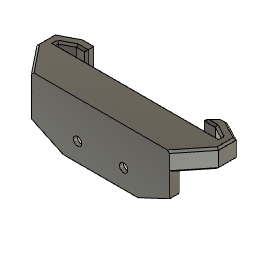
model (Autodesk Fusion 360 design; units mm, degrees)
Autodesk Fusion 360 part; units mm, degrees
sketch "saddle profile" plane through (0, 0, 0) normal (0, 0, 1) x (1, 0, 0) in component "hook"
  line L0 (0, 0) -> (0, 1.45)
  line L1 (0, 1.45) -> (4.9, 4)
  line L2 (4.9, 4) -> (11.5, 4)
  line L3 (11.5, 4) -> (11.5, 8)
  line L4 (11.5, 8) -> (37, 8)
  line L5 (37, 0) -> (0, 0)
  line L6 (37, 8) -> (37, 0) construction
  line L7 (74, 0) -> (74, 1.45)
  line L8 (74, 1.45) -> (69.1, 4)
  line L9 (69.1, 4) -> (62.5, 4)
  line L10 (62.5, 4) -> (62.5, 8)
  line L11 (62.5, 8) -> (37, 8)
  line L12 (37, 0) -> (74, 0)
  line L13 (0, 0) -> (0, -19.5) construction
  line L14 (0, -19.5) -> (74, -19.5) construction
  line L15 (74, -19.5) -> (74, 0) construction
  dimension "d7" = 1.45
  dimension "d8" = 6.6
  dimension "d9" = 4
  dimension "d10" = 11.5
  dimension "d11" = 4
  dimension "d12" = 37
  dimension "d13" = 19.5
  constraint coincident L0.start L5.end
  constraint vertical L0
  constraint perpendicular L0 L2
  constraint perpendicular L2 L3
  constraint perpendicular L3 L4
  constraint perpendicular L0 L5
  constraint perpendicular L5 L6
  constraint symmetric L0.start L6 L7.start
  constraint symmetric L0.end L6 L7.end
  constraint symmetric L1.end L6 L8.end
  constraint symmetric L2.end L6 L9.end
  constraint symmetric L3.end L6 L10.end
  constraint symmetric L4.end L6 L11.end
  constraint symmetric L5.start L6 L12.start
  constraint perpendicular L5 L13
  constraint perpendicular L0 L14
  constraint perpendicular L12 L15
  measures "d7" distance of L0.start L0.end
  measures "d8" distance of L1.end L2.end
  measures "d9" distance of L2 L5
  measures "d10" distance of L0 L3
  measures "d11" distance of L2.end L3.end
  measures "d12" distance of L5.start L0.start
  measures "d13" distance of L0.start L13.end
sketch "mount profile" plane through (0, 0, 0) normal (0, 0, 1) x (1, 0, 0) in component "hook"
  line L0 (-11.6, 4.4845) -> (-11.6, -5)
  line L1 (0, -19.5) -> (74, -19.5)
  line L2 (-6.6, 1.45) -> (-0.1627, 4.8)
  line L3 (5.0442, 9.8) -> (-1.3859, 9.8)
  line L4 (-1.3859, 9.8) -> (-11.6, 4.4845)
  line L5 (-0.1627, 4.8) -> (5.0442, 4.8)
  line L6 (5.0442, 4.8) -> (5.0442, 9.8)
  line L7 (0, 1.45) -> (4.9, 4)
  line L8 (75.3859, 9.8) -> (72.2442, 9.8)
  line L9 (74.1627, 4.8) -> (67.2442, 4.8)
  line L10 (67.2442, 4.8) -> (72.2442, 9.8)
  line L11 (85.6, -5) -> (85.6, 4.4845)
  line L12 (80.6, 0) -> (-6.6, 0)
  line L13 (-6.6, 0) -> (-6.6, 1.45)
  line L14 (80.6, 0) -> (80.6, 1.45)
  line L15 (80.6, 1.45) -> (74.1627, 4.8)
  line L16 (-3.3814, 3.125) -> (-5.6896, 7.5603) construction
  line L17 (85.6, 4.4845) -> (75.3859, 9.8)
  line L18 (77.3814, 3.125) -> (79.6896, 7.5603) construction
  line L19 (85.6, 0.725) -> (80.6, 0.725) construction
  line L20 (-6.6, 0.725) -> (-11.6, 0.725) construction
  line L21 (85.6, -5) -> (74, -19.5)
  line L22 (-11.6, -5) -> (0, -19.5)
  line L23 (85.6, -5) -> (-11.6, -5) construction
  line L24 (37, 0) -> (37, -5) construction
  line L25 (74, -19.5) -> (74, -13.5)
  line L26 (74, -13.5) -> (0, -13.5)
  line L27 (0, -13.5) -> (0, -19.5)
  point P0 (74, 0)
  point P1 (74, -19.5)
  point P2 (0, -19.5)
  dimension "d16" = 74
  dimension "d17" = 1.45
  dimension "d19" = 4.8
  dimension "d20" = 62.2
  dimension "d22" = 6.6
  dimension "d23" = 45
  dimension "d24" = 6.6
  dimension "d25" = 5
  dimension "d26" = 19.5
  dimension "d29" = 6
  dimension "d47" = 5.2069
  constraint vertical L0
  constraint horizontal L1
  constraint parallel L1 L5
  constraint perpendicular L1 L6
  constraint coincident L3.start L6.end
  constraint parallel L2 L7
  constraint coincident L8.end L10.end
  constraint perpendicular L8 L11
  constraint perpendicular L12 L13
  constraint coincident L2.start L13.end
  constraint horizontal L12
  constraint coincident origin L12
  constraint perpendicular L12 L14
  constraint parallel L9 L12
  constraint collinear L5 L9
  constraint equal L13 L14
  constraint equal L2 L15
  constraint parallel L2 L4
  constraint parallel L3 L5
  constraint midpoint L2 L16.start
  constraint coincident L4 L16.end
  constraint perpendicular L4 L16
  constraint equal L6 L16
  constraint collinear L3 L8
  constraint parallel L15 L17
  constraint midpoint L15 L18.start
  constraint coincident L17 L18.end
  constraint perpendicular L17 L18
  constraint equal L6 L18
  constraint coincident L11 L19.start
  constraint midpoint L14 L19.end
  constraint perpendicular L11 L19
  constraint equal L6 L19
  constraint midpoint L13 L20.start
  constraint coincident L0 L20.end
  constraint perpendicular L0 L20
  constraint equal L6 L20
  constraint coincident P1 L1.end
  constraint coincident P2 L1.start
  constraint horizontal L23
  constraint midpoint L12 L24.start
  constraint midpoint L23 L24.end
  constraint equal L6 L24
  constraint perpendicular L1 L25
  constraint perpendicular L25 L26
  constraint perpendicular L1 L27
  measures "d16" distance of L9.end L12.end
  measures "d17" distance of L12.end L2.start
  measures "d19" distance of L9 L12
  measures "d20" distance of L5.end L9.end
  measures "d22" distance of origin L12.end
  measures "d23" angle of L9 L10
  measures "d24" distance of L12.start P0
  measures "d25" distance of L16.start L16.end
  measures "d26" distance of L1 L12
  measures "d29" distance of L1 L26
  measures "d47" distance of L2.end L5.end
extrude "Extrude2" add sketch "mount profile" along normal blind 10 in component "hook"
sketch "mount" plane through (0, -19.5, 0) normal (0, -1, 0) x (1, 0, 0) in component "hook"
  line L0 (0, 0) -> (74, 0)
  line L1 (74, 0) -> (74, 10)
  line L2 (74, 10) -> (0, 10)
  line L3 (0, 10) -> (0, 0)
  line L4 (0, 0) -> (0, -12)
  line L5 (0, -12) -> (17, -20)
  line L6 (17, -20) -> (57, -20)
  line L7 (57, -20) -> (74, -12)
  line L8 (74, -12) -> (74, 0)
  circle A0 centre (24.6397, -10) radius 6.25 construction
  circle A1 centre (49.3603, -10) radius 6.25 construction
  circle A2 centre (24.6397, -10) radius 2.25
  circle A3 centre (49.3603, -10) radius 2.25
  line L9 (24.6397, -10) -> (49.3603, -10) construction
  line L10 (24.6397, -10) -> (0, -12) construction
  line L11 (49.3603, -10) -> (74, -12) construction
  line L12 (42, 0) -> (42, -20)
  line L13 (32, 0) -> (32, -20)
  line L14 (42, -3.75) -> (74, -3.75) construction
  line L15 (32, -3.75) -> (0, -3.75) construction
  dimension "d33" = 12.5
  dimension "d34" = 4.5
  dimension "d35" = 12
  dimension "d36" = 40
  dimension "d37" = 8
  dimension "d40" = 10
  dimension "d42" = 10
  constraint coincident L0.start L3.end
  constraint perpendicular L0 L4
  constraint perpendicular L3 L6
  constraint coincident L0.end L1.start
  constraint parallel L4 L8
  constraint equal L5 L7
  constraint equal L4 L8
  constraint equal A0 A1
  constraint concentric A0 A2
  constraint concentric A1 A3
  constraint equal A2 A3
  constraint coincident A0.centre A2.centre
  constraint coincident A1.centre A3.centre
  constraint horizontal L9
  constraint equal L10 L11
  constraint equal L9 L11
  constraint coincident L0 L12.start
  constraint coincident L6 L12.end
  constraint perpendicular L6 L12
  constraint coincident L0 L13.start
  constraint coincident L6 L13.end
  constraint perpendicular L6 L13
  constraint coincident L12 L14.start
  constraint coincident L8 L14.end
  constraint perpendicular L8 L14
  constraint coincident L13 L15.start
  constraint coincident L4 L15.end
  constraint perpendicular L4 L15
  constraint equal L14 L15
  constraint collinear L14 L15
  constraint tangent A1 L14
  measures "d33" diameter of A0
  measures "d34" diameter of A2
  measures "d35" distance of L0.start L4.end
  measures "d36" distance of L5.end L6.end
  measures "d37" vertical distance of L4.end L5.end
  measures "d40" distance of L6 L9
  measures "d42" distance of L12 L13
extrude "Extrude3" add sketch "mount" against normal blind 6 contours L0 L4 L5 L6 L13 | L0 L6 L12 L13 | L0 L6 L7 L8 L12 in component "hook"
extrude "Extrude4" add sketch "mount" against normal up to surface (13.5 mm away) from surface at -6 contours L0 L6 L12 L13 in component "hook"
chamfer "Chamfer1" distance 4 angle 45 2 edges at (47.2626, -13.5, -10.8136) (22.5419, -13.5, -10.8136) in component "hook"
chamfer "Chamfer2" distance 1 angle 45 47 edges at (74, -13.5, -6) (65.5, -13.5, -16) (49.5, -13.5, -20) (8.5, -13.5, -16) (24.5, -13.5, -20) (0, -13.5, -6) (42, 0, -10) (61.3, 0, 0) (12.7, 0, 0) (32, 0, -10) (37, 0, -20) (42, -6.75, -20) (32, -6.75, -20) (79.8, -12.25, 0) (79.8, -12.25, 10) (85.6, -0.2577, 10) (85.6, -0.2577, 0) (-5.8, -12.25, 0) (-5.8, -12.25, 10) (-11.6, -0.2577, 10) (-11.6, -0.2577, 0) (-6.493, 7.1423, 10) (-6.493, 7.1423, 0) (1.8291, 9.8, 0) (1.8291, 9.8, 10) (5.0442, 9.8, 5) (80.493, 7.1423, 0) (80.493, 7.1423, 10) (73.815, 9.8, 10) (73.815, 9.8, 0) (69.7442, 7.3, 10) (69.7442, 7.3, 0) (5.0442, 4.8, 5) (77.3814, 3.125, 0) (70.7035, 4.8, 0) (80.6, 0.725, 0) (2.4407, 4.8, 0) (-3.3814, 3.125, 0) (-6.6, 0.725, 0) (67.2442, 4.8, 5) (77.3814, 3.125, 10) (37, 0, 10) (80.6, 0.725, 10) (70.7035, 4.8, 10) (2.4407, 4.8, 10) (-3.3814, 3.125, 10) (-6.6, 0.725, 10) in component "hook"
component "hook" placed x (1, 0, 0) y (0, 1, 0) z (0, 0, 1) at (0, 0, 0)
equation "saddleW = 74 mm"
equation "saddleShelfD = 19.5 mm"
equation "saddleLipD = 11.5 mm"
equation "saddleLipT = 4 mm"
equation "saddleLipFlat = 6.6 mm"
equation "saddleEdgeH = 1.45 mm"
equation "d7 = saddleEdgeH"
equation "d8 = saddleLipFlat"
equation "d9 = saddleLipT"
equation "d10 = saddleLipD"
equation "d11 = d9"
equation "d12 = saddleW / 2"
equation "d13 = saddleShelfD"
equation "d16 = saddleW"
equation "d17 = saddleEdgeH"
equation "d19 = saddleLipT * 1.2"
equation "d20 = saddleW - ( 2 * saddleLipD ) + saddleLipFlat + 4.6 mm"
equation "d22 = saddleLipFlat"
equation "d24 = d22"
equation "d26 = saddleShelfD"
equation "mountT = 10 mm"
equation "d31 = mountT"
equation "d42 = mountT"
